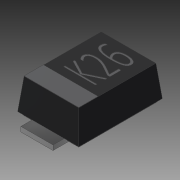
# Autodesk Inventor part: PMEG6020AELR Diode
Saved by Autodesk Inventor 2016 (Build 200138000, 138)
## iProperties
Created: 2019-08-18
Part Number: PMEG6020AELR Diode
Material: Generic
Document SubType Name: Modeling
Designer: Orest
Mass: 0.0048517 g
Surface Area: 0.199036 cm^2
Volume: 0.0048517 cm^3
Density: 1 g/cm^3
Appearance: Smooth - Black (BGA)
Author: Orest
Autodesk Inventor part; units mm, degrees
ref_plane "YZ Plane" through (0, 0, 0) normal (1, 0, 0) x (0, 1, 0)
ref_plane "XZ Plane" through (0, 0, 0) normal (0, 1, 0) x (-1, 0, 0)
sketch "Sketch10" plane through (0, 0, 0) normal (0, 0, 1) x (1, 0, 0)
  line L0 (-1.3, 0.1) -> (-1.2, 1.05)
  line L1 (-1.2, 1.05) -> (1.2, 1.05)
  line L2 (1.2, 1.05) -> (1.3, 0.1)
  line L3 (1.3, 0.1) -> (1.25, 0.1)
  line L4 (1.25, 0.1) -> (1.21, 0)
  line L5 (1.21, 0) -> (-1.21, 0)
  line L6 (-1.21, 0) -> (-1.25, 0.1)
  line L7 (-1.25, 0.1) -> (-1.3, 0.1)
  line L8 (0, 1.05) -> (0, 0) construction
  dimension "d8" = 2.6
  dimension "d9" = 1.05
  dimension "d10" = 0.1
  dimension "d12" = 0.04
  dimension "d13" = 0.05
  dimension "d14" = 0.1
  constraints: 19 end point, 3 parallel, 2 equal length, 2 midpoint, 1 coincident, 1 horizontal, 1 perpendicular, 1 point on line
  measures "d8" distance of L2.end L0.start
  measures "d9" distance between parallel lines of L5 L1
  measures "d10" distance between parallel lines of L5 L7
  measures "d12" horizontal distance of L3.end L4.end
  measures "d13" distance of L6.end L0.start
  measures "d14" horizontal distance of L0.end L0.start
extrude "Extrusion4" add sketch "Sketch10" along normal mid plane 1.9
sketch "Sketch11" plane through (0, 0, 0) normal (1, 0, 0) x (0, 1, 0)
  line L0 (0.1, -0.95) -> (0.1, 0.95) construction
  line L1 (1.05, 0.95) -> (0.1, 0.95) projected
  line L2 (1.05, 0.95) -> (1.05, -0.95) construction
  line L3 (0.1, -0.95) -> (1.05, -0.95) projected
  line L4 (0, -0.95) -> (0, 0.95) construction
  line L5 (0.1, 0.95) -> (0, 0.95) projected
  line L6 (0.1, -0.95) -> (0.1, 0.95) construction
  line L7 (0, -0.95) -> (0.1, -0.95) construction
  line L8 (0.1, 0.95) -> (1.05, 0.85)
  line L9 (0.1, 0.95) -> (0.1, 0.9)
  line L10 (0.1, 0.9) -> (0, 0.86)
  line L11 (1.05, 0) -> (0, 0) construction
  line L12 (1.05, 1) -> (0, 1)
  line L13 (0, 0.86) -> (0, 1)
  line L14 (1.05, 0.85) -> (1.05, 1)
  line L15 (1.05, -0.95) -> (0.1, -0.95)
  line L16 (0.1, -0.95) -> (0, -0.95)
  line L17 (0.1, -0.95) -> (1.05, -0.85)
  line L18 (0.1, -0.95) -> (0.1, -0.9)
  line L19 (0.1, -0.9) -> (0, -0.86)
  line L20 (1.05, -1) -> (0, -1)
  line L21 (0, -0.86) -> (0, -1)
  line L22 (1.05, -0.85) -> (1.05, -1)
  dimension "d18" = 0.1
  dimension "d22" = 0.04
  dimension "d23" = 0.05
  dimension "d24" = 0.15
  constraints: 30 end point, 7 symmetric about line, 3 point on line, 1 collinear, 1 horizontal, 1 midpoint, 1 perpendicular, 1 vertical
  measures "d18" distance from line of L8.end L1
  measures "d22" vertical distance of L9.end L10.end
  measures "d23" distance from line of L5 L9.end
  measures "d24" distance from line of L8.end L12
extrude "Extrusion5" cut sketch "Sketch11" along normal through all both and the other way through all
sketch "Sketch13" plane through (-1.2, 1.05, 0.85) normal (0, 1, 0) x (1, 0, 0)
  line L0 (0, 0) -> (2.4, 0) projected
  line L1 (2.4, 1.7) -> (2.4, 0) construction
  line L2 (2.4, 1.7) -> (0, 1.7) construction
  line L3 (0, 0) -> (0, 1.7) projected
  line L4 (0.6, 0) -> (0, 0)
  line L5 (0, 0) -> (0, 1.7)
  line L6 (0, 1.7) -> (0.6, 1.7)
  line L7 (0.6, 1.7) -> (0.6, 0)
  line L8 (0.6, 1.7) -> (2.4, 1.7) construction
  line L9 (2.4, 1.7) -> (2.4, 0) construction
  line L10 (2.4, 0) -> (0.6, 0) construction
  line L11 (0.6, 0) -> (0.6, 1.7) construction
  spline S0 degree 2 poles (1.2338, 0.3692) (1.2338, 0.3636) (1.2319, 0.3561) (1.2254, 0.3505) (1.2141, 0.3477) (1.2056, 0.3477) knots 0 0 0 1 2 3 4 4 4
  spline S1 degree 2 poles (1.2056, 0.3477) (1.1972, 0.3477) (1.1803, 0.3505) (1.1709, 0.3608) (1.1681, 0.3674) knots 0 0 0 1 2 3 3 3
  line L12 (1.1681, 0.3674) -> (0.9268, 0.8782)
  line L13 (0.9268, 0.8782) -> (0.9268, 0.3674)
  spline S2 degree 2 poles (0.9268, 0.3674) (0.9268, 0.3627) (0.9239, 0.3552) (0.9174, 0.3505) (0.907, 0.3477) (0.8986, 0.3477) knots 0 0 0 1 2 3 4 4 4
  spline S3 degree 2 poles (0.8986, 0.3477) (0.8901, 0.3477) (0.8798, 0.3505) (0.8732, 0.3552) (0.8704, 0.3627) (0.8704, 0.3674) knots 0 0 0 1 2 3 4 4 4
  line L14 (0.8704, 0.3674) -> (0.8704, 1.3326)
  spline S4 degree 2 poles (0.8704, 1.3326) (0.8704, 1.3373) (0.8732, 1.3448) (0.8798, 1.3495) (0.8901, 1.3523) (0.8986, 1.3523) knots 0 0 0 1 2 3 4 4 4
  spline S5 degree 2 poles (0.8986, 1.3523) (0.907, 1.3523) (0.9174, 1.3495) (0.9239, 1.3448) (0.9268, 1.3373) (0.9268, 1.3326) knots 0 0 0 1 2 3 4 4 4
  line L15 (0.9268, 1.3326) -> (0.9268, 0.88)
  line L16 (0.9268, 0.88) -> (1.1577, 1.3326)
  spline S6 degree 2 poles (1.1577, 1.3326) (1.1606, 1.3383) (1.1671, 1.3458) (1.1756, 1.3505) (1.1859, 1.3523) (1.1944, 1.3523) knots 0 0 0 1 2 3 4 4 4
  spline S7 degree 2 poles (1.1944, 1.3523) (1.2028, 1.3523) (1.2131, 1.3495) (1.2188, 1.3439) (1.2207, 1.3373) (1.2207, 1.3326) knots 0 0 0 1 2 3 4 4 4
  spline S8 degree 2 poles (1.2207, 1.3326) (1.2207, 1.3242) (1.216, 1.3082) (1.2094, 1.2979) knots 0 0 0 1 2 2 2
  line L17 (1.2094, 1.2979) -> (0.9925, 0.8829)
  line L18 (0.9925, 0.8829) -> (1.2244, 0.3974)
  spline S9 degree 2 poles (1.2244, 0.3974) (1.231, 0.3843) (1.2338, 0.373) (1.2338, 0.3692) knots 0 0 0 1 2 2 2
  spline S10 degree 2 poles (1.6779, 0.3955) (1.6779, 0.3862) (1.6751, 0.3702) (1.6714, 0.3589) (1.6648, 0.3523) (1.6601, 0.3523) knots 0 0 0 1 2 3 4 4 4
  line L19 (1.6601, 0.3523) -> (1.338, 0.3523)
  spline S11 degree 2 poles (1.338, 0.3523) (1.3343, 0.3523) (1.3268, 0.357) (1.3211, 0.3674) (1.3183, 0.3843) (1.3183, 0.3955) knots 0 0 0 1 2 3 4 4 4
  spline S12 degree 2 poles (1.3183, 0.3955) (1.3183, 0.4059) (1.3192, 0.4209) (1.3221, 0.4331) (1.3268, 0.4453) (1.3305, 0.4528) knots 0 0 0 1 2 3 4 4 4
  line L20 (1.3305, 0.4528) -> (1.4526, 0.6678)
  spline S13 degree 2 poles (1.4526, 0.6678) (1.4977, 0.7477) (1.5521, 0.8744) (1.5803, 0.9758) (1.5897, 1.0585) (1.5897, 1.0951) knots 0 0 0 1 2 3 4 4 4
  spline S14 degree 2 poles (1.5897, 1.0951) (1.5897, 1.1326) (1.5746, 1.1993) (1.5474, 1.2491) (1.5061, 1.2791) (1.4798, 1.2791) knots 0 0 0 1 2 3 4 4 4
  spline S15 degree 2 poles (1.4798, 1.2791) (1.4507, 1.2791) (1.4047, 1.2528) (1.37, 1.219) (1.3465, 1.1927) (1.3408, 1.1927) knots 0 0 0 1 2 3 4 4 4
  spline S16 degree 2 poles (1.3408, 1.1927) (1.338, 1.1927) (1.3343, 1.1974) (1.3305, 1.2068) (1.3296, 1.2228) (1.3296, 1.2322) knots 0 0 0 1 2 3 4 4 4
  spline S17 degree 2 poles (1.3296, 1.2322) (1.3296, 1.2415) (1.3305, 1.2538) (1.3324, 1.2641) (1.3352, 1.2735) (1.3455, 1.2885) (1.3709, 1.3148) (1.4103, 1.342) (1.4573, 1.3608) (1.4826, 1.3608) knots 0 0 0 1 2 3 4 5 6 7 8 8 8
  spline S18 degree 2 poles (1.4826, 1.3608) (1.5239, 1.3608) (1.5869, 1.3195) (1.6282, 1.2491) (1.6488, 1.1552) (1.6488, 1.1035) knots 0 0 0 1 2 3 4 4 4
  spline S19 degree 2 poles (1.6488, 1.1035) (1.6488, 1.0566) (1.6385, 0.9617) (1.6066, 0.85) (1.5465, 0.7148) (1.4958, 0.6265) knots 0 0 0 1 2 3 4 4 4
  line L21 (1.4958, 0.6265) -> (1.3878, 0.4359)
  line L22 (1.3878, 0.4359) -> (1.6601, 0.4359)
  spline S20 degree 2 poles (1.6601, 0.4359) (1.6638, 0.4359) (1.6704, 0.4312) (1.6751, 0.42) (1.6779, 0.4049) (1.6779, 0.3955) knots 0 0 0 1 2 3 4 4 4
  spline S21 degree 2 poles (2.1746, 0.6697) (2.1746, 0.6096) (2.1531, 0.4904) (2.1052, 0.3974) (2.0291, 0.3392) (1.9765, 0.3392) knots 0 0 0 1 2 3 4 4 4
  spline S22 degree 2 poles (1.9765, 0.3392) (1.9418, 0.3392) (1.8873, 0.3692) (1.846, 0.4256) (1.8178, 0.5082) (1.8009, 0.6143) (1.7925, 0.7411) (1.7925, 0.8143) knots 0 0 0 1 2 3 4 5 6 6 6
  spline S23 degree 2 poles (1.7925, 0.8143) (1.7925, 0.881) (1.8019, 1.0143) (1.8244, 1.1345) (1.861, 1.2397) (1.9155, 1.3157) (1.9887, 1.3599) (2.0376, 1.3599) knots 0 0 0 1 2 3 4 5 6 6 6
  spline S24 degree 2 poles (2.0376, 1.3599) (2.0545, 1.3599) (2.0883, 1.3523) (2.1174, 1.342) (2.1371, 1.3279) (2.1437, 1.3195) (2.1465, 1.311) (2.1484, 1.3016) (2.1493, 1.2904) (2.1493, 1.2829) knots 0 0 0 1 2 3 4 5 6 7 8 8 8
  spline S25 degree 2 poles (2.1493, 1.2829) (2.1493, 1.2744) (2.1493, 1.2603) (2.1465, 1.2509) (2.1418, 1.2453) (2.138, 1.2453) knots 0 0 0 1 2 3 4 4 4
  spline S26 degree 2 poles (2.138, 1.2453) (2.1333, 1.2453) (2.1164, 1.2566) (2.0911, 1.2697) (2.0545, 1.281) (2.03, 1.281) knots 0 0 0 1 2 3 4 4 4
  spline S27 degree 2 poles (2.03, 1.281) (1.984, 1.281) (1.9174, 1.2162) (1.8732, 1.1073) (1.8526, 0.9636) (1.8507, 0.8857) knots 0 0 0 1 2 3 4 4 4
  spline S28 degree 2 poles (1.8507, 0.8857) (1.8638, 0.8979) (1.8958, 0.9223) (1.9333, 0.942) (1.9756, 0.9542) (2, 0.9542) knots 0 0 0 1 2 3 4 4 4
  spline S29 degree 2 poles (2, 0.9542) (2.0498, 0.9542) (2.1174, 0.9092) (2.1577, 0.8312) (2.1746, 0.7279) (2.1746, 0.6697) knots 0 0 0 1 2 3 4 4 4
  spline S30 degree 2 poles (2.1155, 0.6603) (2.1155, 0.7082) (2.1042, 0.789) (2.0751, 0.8453) (2.0272, 0.8772) (1.9925, 0.8772) knots 0 0 0 1 2 3 4 4 4
  spline S31 degree 2 poles (1.9925, 0.8772) (1.9737, 0.8772) (1.9343, 0.866) (1.8977, 0.8453) (1.8648, 0.819) (1.8516, 0.8031) knots 0 0 0 1 2 3 4 4 4
  spline S32 degree 2 poles (1.8516, 0.8031) (1.8516, 0.6951) (1.8695, 0.5486) (1.9023, 0.4585) (1.9512, 0.419) (1.984, 0.419) knots 0 0 0 1 2 3 4 4 4
  spline S33 degree 2 poles (1.984, 0.419) (2.0188, 0.419) (2.0685, 0.4631) (2.1005, 0.5336) (2.1155, 0.6181) (2.1155, 0.6603) knots 0 0 0 1 2 3 4 4 4
  point P0 (1.2, 0.85)
  dimension "d26" = 0.6
  constraints: 8 end point, 7 collinear, 2 parallel, 1 horizontal, 1 perpendicular, 2 other
  measures "d26" distance between parallel lines of L7 L5
extrude "Extrusion6" cut sketch "Sketch13" against normal blind 0.01 contours L13 S2 S3 L14 S4 S5 L15 | S0 S1 L12 L16 S6 S7 S8 L17 L18 S9 | S10 L19 S11 S12 L20 S13 S14 S15 S16 S17 S18 S19 L21 L22 S20 | S21 S22 S23 S24 S25 S26 S27 S28 S29
extrude "Extrusion7" add sketch "Sketch13" along normal blind 0.01 contours L3 L6 L7 L0
ref_plane "Work Plane1" through (-1.21, -0.05, 0.86) normal (0, -1, 0) x (1, 0, 0)
sketch "Sketch14" plane through (-1.21, -0.05, 0.86) normal (0, -1, 0) x (1, 0, 0)
  line L0 (0.06, -0.36) -> (-0.44, -0.36)
  line L1 (-0.44, -0.36) -> (-0.44, -1.36)
  line L2 (-0.44, -1.36) -> (0.06, -1.36)
  line L3 (0.06, -1.36) -> (0.06, -0.36)
  line L4 (2.36, -0.36) -> (2.86, -0.36)
  line L5 (2.86, -0.36) -> (2.86, -1.36)
  line L6 (2.86, -1.36) -> (2.36, -1.36)
  line L7 (2.36, -1.36) -> (2.36, -0.36)
  line L8 (2.42, 0) -> (0, 0) construction
  line L9 (0, -1.72) -> (0, 0) construction
  line L10 (0, -1.72) -> (2.42, -1.72) construction
  line L11 (2.42, -1.72) -> (2.42, 0) construction
  line L12 (0.06, -0.86) -> (2.36, -0.86) construction
  point P0 (1.21, -0.86)
  point P1 (1.21, -0.86)
  dimension "d32" = 3.3
  dimension "d33" = 1
  dimension "d34" = 2.3
  constraints: 18 end point, 4 parallel, 3 collinear, 3 midpoint, 2 horizontal, 2 perpendicular, 1 coincident
  measures "d32" distance between parallel lines of L5 L1
  measures "d33" distance between parallel lines of L2 L0
  measures "d34" distance between parallel lines of L7 L3
extrude "Extrusion8" add sketch "Sketch14" against normal up to surface (0.15 mm away)
equation "\"d18\" = d14"
equation "\"d22\" = d12"
equation "\"d23\" = d13"
body "Solid4"
